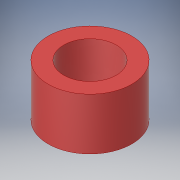
# Autodesk Inventor part: retention_auger_ring
Saved by Autodesk Inventor 2019 (Build 230136000, 136)
## iProperties
Created: 2019-05-07
Part Number: retention_auger_ring
Material: Generic
Document SubType Name: Modeling
Designer: assman
Density: 1 g/cm^3
Appearance: Smooth - Red
Author: assman
## iProperties of the stored document retention_auger_ring_3DPrint.ipt
Created: 2019-05-07
Part Number: retention_auger_ring_3DPrint
Material: Generic
Document SubType Name: Modeling
Designer: assman
Density: 1 g/cm^3
Appearance: Default
Author: assman
Autodesk Inventor part; units mm, degrees
ref_plane "YZ Plane" through (0, 0, 0) normal (1, 0, 0) x (0, 1, 0)
ref_plane "XZ Plane" through (0, 0, 0) normal (0, 1, 0) x (-1, 0, 0)
ref_plane "XY Plane" through (0, 0, 0) normal (0, 0, 1) x (1, 0, 0)
sketch "Sketch1" plane through (0, 0, 0) normal (0, 1, 0) x (-1, 0, 0)
  circle A0 centre (0, 0) radius 4.9855 construction
  circle A1 centre (0, 0) radius 5.0655
  circle A2 centre (0, 0) radius 5.0655
  circle A3 centre (0, 0) radius 8.0655
  dimension "d0" = 9.971
  dimension "d1" = 0.08
  dimension "d2" = 3
  constraints: 4 centre point, 2 coincident, 1 concentric
  measures "d0" diameter of A0
  measures "d1" radial gap between concentric circles of A0 A1
  measures "d2" radial gap between concentric circles of A1 A3
extrude "Extrusion1" add sketch "Sketch1" along normal blind 10
body "Solid1"
